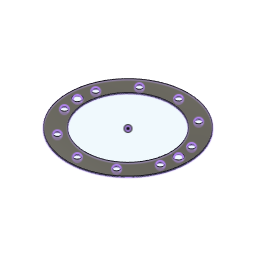
fotobox controller (Autodesk Fusion 360 design; units mm, degrees)
Autodesk Fusion 360 part; units mm, degrees
note: some values were not read from the file. Set by a fixed rule: which sketch regions a step uses.
sketch "Skizze1" plane through (0, 0, 0) normal (0, 0, 1) x (1, 0, 0)
  circle A0 centre (0, 0) radius 45 construction
  circle A1 centre (0, 0) radius 47.5
  circle A2 centre (0, 0) radius 55 construction
  line L0 (2.6555, 52.4998) -> (-2.3445, 52.4998)
  line L1 (-2.3445, 52.4998) -> (-2.3445, 57.4998)
  line L2 (-2.3445, 57.4998) -> (2.6555, 57.4998)
  line L3 (2.6555, 57.4998) -> (2.6555, 52.4998)
  line L4 (2.6555, 52.4998) -> (-2.3445, 57.4998) construction
  line L5 (-2.3445, 52.4998) -> (2.6555, 57.4998) construction
  line L6 (-31.6491, 48.0792) -> (-28.7102, 44.0341)
  line L7 (-28.7102, 44.0341) -> (-32.7553, 41.0952)
  line L8 (-32.7553, 41.0952) -> (-35.6942, 45.1403)
  line L9 (-35.6942, 45.1403) -> (-31.6491, 48.0792)
  line L10 (-53.8649, 20.294) -> (-49.1096, 18.7489)
  line L11 (-49.1096, 18.7489) -> (-50.6547, 13.9936)
  line L12 (-50.6547, 13.9936) -> (-55.41, 15.5387)
  line L13 (-55.41, 15.5387) -> (-53.8649, 20.294)
  line L14 (-55.5062, -15.2428) -> (-50.7509, -13.6977)
  line L15 (-50.7509, -13.6977) -> (-49.2058, -18.453)
  line L16 (-49.2058, -18.453) -> (-53.9611, -19.9981)
  line L17 (-53.9611, -19.9981) -> (-55.5062, -15.2428)
  line L18 (-35.9459, -44.9574) -> (-33.007, -40.9123)
  line L19 (-33.007, -40.9123) -> (-28.9619, -43.8512)
  line L20 (-28.9619, -43.8512) -> (-31.9008, -47.8963)
  line L21 (-31.9008, -47.8963) -> (-35.9459, -44.9574)
  line L22 (-2.6555, -57.4998) -> (-2.6555, -52.4998)
  line L23 (-2.6555, -52.4998) -> (2.3445, -52.4998)
  line L24 (2.3445, -52.4998) -> (2.3445, -57.4998)
  line L25 (2.3445, -57.4998) -> (-2.6555, -57.4998)
  line L26 (31.6491, -48.0792) -> (28.7102, -44.0341)
  line L27 (28.7102, -44.0341) -> (32.7553, -41.0952)
  line L28 (32.7553, -41.0952) -> (35.6942, -45.1403)
  line L29 (35.6942, -45.1403) -> (31.6491, -48.0792)
  line L30 (53.8649, -20.294) -> (49.1096, -18.7489)
  line L31 (49.1096, -18.7489) -> (50.6547, -13.9936)
  line L32 (50.6547, -13.9936) -> (55.41, -15.5387)
  line L33 (55.41, -15.5387) -> (53.8649, -20.294)
  line L34 (55.5062, 15.2428) -> (50.7509, 13.6977)
  line L35 (50.7509, 13.6977) -> (49.2058, 18.453)
  line L36 (49.2058, 18.453) -> (53.9611, 19.9981)
  line L37 (53.9611, 19.9981) -> (55.5062, 15.2428)
  line L38 (35.9459, 44.9574) -> (33.007, 40.9123)
  line L39 (33.007, 40.9123) -> (28.9619, 43.8512)
  line L40 (28.9619, 43.8512) -> (31.9008, 47.8963)
  line L41 (31.9008, 47.8963) -> (35.9459, 44.9574)
  circle A3 centre (0, 0) radius 62.5
  line L42 (-62.5, 30) -> (-102.5, 30)
  line L43 (-102.5, 30) -> (-102.5, -30)
  line L44 (-102.5, -30) -> (-62.5, -30)
  line L45 (-62.5, -30) -> (-62.5, 30)
  line L46 (-102.5, 0) -> (-62.5, 0) construction
  line L47 (-62.5, -30) -> (-54.8293, -30)
  line L48 (-62.5, 30) -> (-54.8293, 30)
  circle A4 centre (55, 0) radius 2.5
  circle A5 centre (-55, 0) radius 2.5
  point P0 (0.1555, 54.9998)
  dimension "d1" = 90
  dimension "d2" = 2.5
  dimension "d3" = 5
  dimension "d4" = 5
  dimension "d6" = 360
  dimension "d7" = 110
  dimension "d8" = 125
  dimension "d9" = 40
  dimension "d10" = 60
  dimension "d16" = 5
  dimension "d18" = 5
  dimension "d19" = 110
  constraint coincident A0.centre A1.centre
  constraint perpendicular L0 L1
  constraint parallel L0 L2
  constraint parallel L1 L3
  constraint coincident L4 P0
  constraint coincident L5 P0
  constraint coincident A2 P0
  constraint horizontal L0
  constraint concentric A2 A3
  constraint horizontal L42
  constraint vertical L43
  constraint horizontal L44
  constraint vertical L45
  constraint tangent A3 L45
  constraint midpoint L43 L46.start
  constraint midpoint L45 L46.end
  constraint coincident A0.centre L46
  constraint coincident A3 L47.end
  constraint perpendicular L45 L47
  constraint coincident A3 L48.end
  constraint perpendicular L45 L48
  constraint coincident A2 A4.centre
  constraint coincident A2 A5.centre
  constraint horizontal A4.centre A5.centre
  measures "d1" diameter of A0
  measures "d3" distance of L1.end L2.end
  measures "d4" distance of L0.end L1.end
  measures "d7" diameter of A2
  measures "d8" diameter of A3
  measures "d9" distance of L42.start L42.end
  measures "d10" distance of L42.end L43.end
  measures "d16" diameter of A4
  measures "d18" diameter of A5
  measures "d19" distance of A4.centre A5.centre
extrude "Extrusion1" add sketch "Skizze1" along normal blind 1.6 makes body 1
fillet "Abrundung1" radius 10 2 edges at (-54.8293, 30, 0.8) (-54.8293, -30, 0.8) on bodies 1
sketch "Skizze2" plane through (0, 0, 1.6) normal (0, 0, 1) x (-1, 0, 0)
  circle A0 centre (0, 0) radius 47.5
  line L0 (-28.9619, -43.8512) -> (-31.9008, -47.8963)
  line L1 (-31.9008, -47.8963) -> (-35.9459, -44.9574)
  line L2 (-35.9459, -44.9574) -> (-33.007, -40.9123)
  line L3 (-33.007, -40.9123) -> (-28.9619, -43.8512)
  line L4 (-49.2058, -18.453) -> (-53.9611, -19.9981)
  line L5 (-53.9611, -19.9981) -> (-55.5062, -15.2428)
  line L6 (-55.5062, -15.2428) -> (-50.7509, -13.6977)
  line L7 (-50.7509, -13.6977) -> (-49.2058, -18.453)
  line L8 (-50.6547, 13.9936) -> (-55.41, 15.5387)
  line L9 (-55.41, 15.5387) -> (-53.8649, 20.294)
  line L10 (-53.8649, 20.294) -> (-49.1096, 18.7489)
  line L11 (-49.1096, 18.7489) -> (-50.6547, 13.9936)
  line L12 (-32.7553, 41.0952) -> (-35.6942, 45.1403)
  line L13 (-35.6942, 45.1403) -> (-31.6491, 48.0792)
  line L14 (-31.6491, 48.0792) -> (-28.7102, 44.0341)
  line L15 (-28.7102, 44.0341) -> (-32.7553, 41.0952)
  line L16 (-2.3445, 52.4998) -> (-2.3445, 57.4998)
  line L17 (-2.3445, 57.4998) -> (2.6555, 57.4998)
  line L18 (2.6555, 57.4998) -> (2.6555, 52.4998)
  line L19 (2.6555, 52.4998) -> (-2.3445, 52.4998)
  line L20 (28.9619, 43.8512) -> (31.9008, 47.8963)
  line L21 (31.9008, 47.8963) -> (35.9459, 44.9574)
  line L22 (35.9459, 44.9574) -> (33.007, 40.9123)
  line L23 (33.007, 40.9123) -> (28.9619, 43.8512)
  line L24 (49.2058, 18.453) -> (53.9611, 19.9981)
  line L25 (53.9611, 19.9981) -> (55.5062, 15.2428)
  line L26 (55.5062, 15.2428) -> (50.7509, 13.6977)
  line L27 (50.7509, 13.6977) -> (49.2058, 18.453)
  line L28 (50.6547, -13.9936) -> (55.41, -15.5387)
  line L29 (55.41, -15.5387) -> (53.8649, -20.294)
  line L30 (53.8649, -20.294) -> (49.1096, -18.7489)
  line L31 (49.1096, -18.7489) -> (50.6547, -13.9936)
  line L32 (32.7553, -41.0952) -> (35.6942, -45.1403)
  line L33 (35.6942, -45.1403) -> (31.6491, -48.0792)
  line L34 (31.6491, -48.0792) -> (28.7102, -44.0341)
  line L35 (28.7102, -44.0341) -> (32.7553, -41.0952)
  line L36 (2.3445, -57.4998) -> (-2.6555, -57.4998)
  line L37 (-2.6555, -57.4998) -> (-2.6555, -52.4998)
  line L38 (-2.6555, -52.4998) -> (2.3445, -52.4998)
  line L39 (2.3445, -52.4998) -> (2.3445, -57.4998)
  line L40 (102.5, -30) -> (102.5, 30)
  line L41 (102.5, 30) -> (60.4669, 30)
  arc A1 (52.1267, 34.4828) -> (60.4669, 30) centre (60.4669, 40) ccw
  arc A2 (52.1267, 34.4828) -> (52.1267, -34.4828) centre (0, 0) ccw
  arc A3 (60.4669, -30) -> (52.1267, -34.4828) centre (60.4669, -40) ccw
  line L42 (60.4669, -30) -> (102.5, -30)
  circle A4 centre (55, 0) radius 2.5
  circle A5 centre (-55, 0) radius 2.5
sketch "Skizze1 (2)" plane through (0, 0, 0) normal (0, 0, 1) x (1, 0, 0) in component "Blende"
  circle A0 centre (0, 0) radius 47.5
  circle A1 centre (55, 0) radius 2.5
  circle A2 centre (-55, 0) radius 2.5
  line L0 (-50.7509, -13.6977) -> (-49.2058, -18.453) construction
  line L1 (-49.2058, -18.453) -> (-53.9611, -19.9981) construction
  line L2 (-55.5062, -15.2428) -> (-50.7509, -13.6977) construction
  line L3 (-53.9611, -19.9981) -> (-55.5062, -15.2428) construction
  line L4 (-31.9008, -47.8963) -> (-35.9459, -44.9574) construction
  line L5 (-35.9459, -44.9574) -> (-33.007, -40.9123) construction
  line L6 (-28.9619, -43.8512) -> (-31.9008, -47.8963) construction
  line L7 (-33.007, -40.9123) -> (-28.9619, -43.8512) construction
  line L8 (2.3445, -57.4998) -> (-2.6555, -57.4998) construction
  line L9 (-2.6555, -57.4998) -> (-2.6555, -52.4998) construction
  line L10 (2.3445, -52.4998) -> (2.3445, -57.4998) construction
  line L11 (-2.6555, -52.4998) -> (2.3445, -52.4998) construction
  line L12 (35.6942, -45.1403) -> (31.6491, -48.0792) construction
  line L13 (31.6491, -48.0792) -> (28.7102, -44.0341) construction
  line L14 (32.7553, -41.0952) -> (35.6942, -45.1403) construction
  line L15 (28.7102, -44.0341) -> (32.7553, -41.0952) construction
  line L16 (55.41, -15.5387) -> (53.8649, -20.294) construction
  line L17 (53.8649, -20.294) -> (49.1096, -18.7489) construction
  line L18 (50.6547, -13.9936) -> (55.41, -15.5387) construction
  line L19 (49.1096, -18.7489) -> (50.6547, -13.9936) construction
  line L20 (53.9611, 19.9981) -> (55.5062, 15.2428) construction
  line L21 (55.5062, 15.2428) -> (50.7509, 13.6977) construction
  line L22 (49.2058, 18.453) -> (53.9611, 19.9981) construction
  line L23 (50.7509, 13.6977) -> (49.2058, 18.453) construction
  line L24 (33.007, 40.9123) -> (28.9619, 43.8512) construction
  line L25 (28.9619, 43.8512) -> (31.9008, 47.8963) construction
  line L26 (35.9459, 44.9574) -> (33.007, 40.9123) construction
  line L27 (31.9008, 47.8963) -> (35.9459, 44.9574) construction
  line L28 (2.6555, 52.4998) -> (-2.3445, 52.4998) construction
  line L29 (-2.3445, 52.4998) -> (-2.3445, 57.4998) construction
  line L30 (2.6555, 57.4998) -> (2.6555, 52.4998) construction
  line L31 (-2.3445, 57.4998) -> (2.6555, 57.4998) construction
  line L32 (-28.7102, 44.0341) -> (-32.7553, 41.0952) construction
  line L33 (-32.7553, 41.0952) -> (-35.6942, 45.1403) construction
  line L34 (-31.6491, 48.0792) -> (-28.7102, 44.0341) construction
  line L35 (-35.6942, 45.1403) -> (-31.6491, 48.0792) construction
  line L36 (-49.1096, 18.7489) -> (-50.6547, 13.9936) construction
  line L37 (-50.6547, 13.9936) -> (-55.41, 15.5387) construction
  line L38 (-53.8649, 20.294) -> (-49.1096, 18.7489) construction
  line L39 (-55.41, 15.5387) -> (-53.8649, 20.294) construction
  circle A3 centre (0, 0) radius 65
  circle A4 centre (-55, 0) radius 4
  circle A5 centre (55, 0) radius 4
  circle A6 centre (-0.1555, -54.9998) radius 3
  circle A7 centre (32.2022, -44.5872) radius 3
  circle A8 centre (52.2598, -17.1438) radius 3
  circle A9 centre (52.356, 16.8479) radius 3
  circle A10 centre (32.4539, 44.4043) radius 3
  circle A11 centre (0.1555, 54.9998) radius 3
  circle A12 centre (-32.2022, 44.5872) radius 3
  circle A13 centre (-52.2598, 17.1438) radius 3
  circle A14 centre (-52.356, -16.8479) radius 3
  circle A15 centre (-32.4539, -44.4043) radius 3
  dimension "d20" = 130
  dimension "d29" = 8
  dimension "d30" = 8
  dimension "d32" = 6
  dimension "d34" = 360
  constraint concentric A0 A3
  constraint concentric A2 A4
  constraint concentric A1 A5
  measures "d20" diameter of A3
  measures "d29" diameter of A4
  measures "d30" diameter of A5
  measures "d32" diameter of A6
extrude "Extrusion1'" add sketch "Skizze1 (2)" along normal blind 2 separate body contours A1 | A2 | A3 | A4 | A5 makes body 2 in component "Blende"
extrude "Extrusion2" add sketch "Skizze1 (2)" against normal blind 4 contours A1 | A2 | A4 | A5 bodies 2 in component "Blende"
sketch "Skizze2 (2)" plane through (0, 0, -4) normal (0, 0, -1) x (1, 0, 0) in component "Blende"
  circle A0 centre (55, 0) radius 2.4
  circle A1 centre (-55, 0) radius 2.4
  circle A2 centre (55, 0) radius 4
  circle A3 centre (-55, 0) radius 4
  dimension "d25" = 4.8
  dimension "d26" = 4.8
  measures "d25" diameter of A0
  measures "d26" diameter of A1
extrude "Extrusion3" cut sketch "Skizze2 (2)" against normal up to surface (5 mm away) contours A0 | A1 bodies 2 in component "Blende"
chamfer "Fase1" distance 0.5 angle 45 10 edges at (29.6569, 45.4892, 2) (-2.6414, 56.0846, 2) (-34.9992, 45.672, 2) (-55.0568, 18.2286, 2) (-55.1529, -15.7631, 2) (49.559, 17.9328, 2) (49.4629, -16.059, 2) (29.4052, -43.5023, 2) (-2.9525, -53.9149, 2) (-35.2509, -43.3195, 2) on bodies 2 in component "Blende"
sketch "Skizze5" plane through (0, 0, 2) normal (0, 0, 1) x (-1, 0, 0) in component "Blende"
  circle A0 centre (0.1555, 54.9998) radius 3.5
  circle A1 centre (-52.2598, 17.1438) radius 3.5
  circle A2 centre (52.356, 16.8479) radius 3.5
  circle A3 centre (32.2022, -44.5872) radius 3.5
  circle A4 centre (-32.4539, -44.4043) radius 3.5
  circle A5 centre (0, 0) radius 47.5
  circle A6 centre (0, 0) radius 65
  circle A7 centre (-0.1555, -54.9998) radius 3.5
  circle A8 centre (52.2598, -17.1438) radius 3.5
  circle A9 centre (-52.356, -16.8479) radius 3.5
  circle A10 centre (-32.2022, 44.5872) radius 3.5
  circle A11 centre (32.4539, 44.4043) radius 3.5
  circle A12 centre (0, 0) radius 44.5
  circle A13 centre (0, 0) radius 42.5
  dimension "d37" = -3
  dimension "d38" = -5
extrude "Extrusion4" add sketch "Skizze5" against normal up to surface (2 mm away) contours A5 | A12 bodies 2 in component "Blende"
extrude "Extrusion5" add sketch "Skizze5" against normal blind 8 contours A12 bodies 2 in component "Blende"
chamfer "Fase2" distance 1.5 angle 45 1 edges at (-60.6013, -23.505, 2) on bodies 2 in component "Blende"
chamfer "Fase3" distance 1 angle 45 1 edges at (39.6239, -15.3687, 2) on bodies 2 in component "Blende"
fillet "Abrundung1'" radius 1 1 edges at (41.4886, 16.0919, 0) on bodies 2 in component "Blende"
sketch "Skizze6" plane through (0, 0, 0) normal (0, 0, 1) x (1, 0, 0) in component "Blende"
  circle A0 centre (0, 0) radius 65
  circle A1 centre (-52.2598, 17.1438) radius 3 construction
  circle A2 centre (-52.356, -16.8479) radius 3 construction
  circle A3 centre (-32.2022, 44.5872) radius 3 construction
  circle A4 centre (0.1555, 54.9998) radius 3 construction
  circle A5 centre (32.4539, 44.4043) radius 3 construction
  circle A6 centre (52.356, 16.8479) radius 3 construction
  circle A7 centre (52.2598, -17.1438) radius 3 construction
  circle A8 centre (32.2022, -44.5872) radius 3 construction
  circle A9 centre (-0.1555, -54.9998) radius 3 construction
  circle A10 centre (-32.4539, -44.4043) radius 3 construction
  circle A11 centre (-55, 0) radius 4 construction
  circle A12 centre (55, 0) radius 4 construction
  circle A13 centre (0, 0) radius 47.5 construction
  circle A14 centre (-0.1555, -54.9998) radius 3.5
  circle A15 centre (32.2022, -44.5872) radius 3.5
  circle A16 centre (52.2598, -17.1438) radius 3.5
  circle A17 centre (52.356, 16.8479) radius 3.5
  circle A18 centre (32.4539, 44.4043) radius 3.5
  circle A19 centre (0.1555, 54.9998) radius 3.5
  circle A20 centre (-32.2022, 44.5872) radius 3.5
  circle A21 centre (-52.2598, 17.1438) radius 3.5
  circle A22 centre (-52.356, -16.8479) radius 3.5
  circle A23 centre (-32.4539, -44.4043) radius 3.5
  circle A24 centre (55, 0) radius 4.5
  circle A25 centre (-55, 0) radius 4.5
  circle A26 centre (0, 0) radius 46.5
  dimension "d47" = 7
  dimension "d49" = 360
  dimension "d50" = 9
  dimension "d51" = 9
  dimension "d52" = -1
  constraint concentric A9 A14
  constraint concentric A12 A24
  constraint concentric A11 A25
  measures "d47" diameter of A14
  measures "d50" diameter of A24
  measures "d51" diameter of A25
extrude "Extrusion6" add sketch "Skizze6" along normal blind 1 separate body makes body 3 in component "Blende"
sketch "Skizze7" plane through (0, 0, 0) normal (0, 0, -1) x (1, 0, 0) in component "Blende"
  circle A0 centre (52.356, -16.8479) radius 3.5
  circle A1 centre (32.4539, -44.4043) radius 3.5
  circle A2 centre (-52.2598, -17.1438) radius 3.5
  circle A3 centre (-32.2022, -44.5872) radius 3.5
  circle A4 centre (0.1555, -54.9998) radius 3.5
  circle A5 centre (-52.356, 16.8479) radius 3.5
  circle A6 centre (-32.4539, 44.4043) radius 3.5
  circle A7 centre (55, 0) radius 4.5
  circle A8 centre (-55, 0) radius 4.5
  circle A9 centre (0, 0) radius 46.5
  circle A10 centre (52.2598, 17.1438) radius 3.5
  circle A11 centre (32.2022, 44.5872) radius 3.5
  circle A12 centre (-0.1555, 54.9998) radius 3.5
  circle A13 centre (0, 0) radius 65
component "Blende" placed x (1, 0, 0) y (0, 1, 0) z (0, 0, 1) at (0, 0, 0)
hidden bodies 2
equation "d26 = d25"
equation "d29 = d30"
equation "d38 = d37 - 2 mm"
named bodies: "blende", "DXF Fraese"
